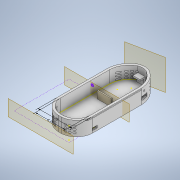
# Autodesk Inventor part: SkateBodyV2
Saved by Autodesk Inventor 2022 (Build 260153000, 153)
## iProperties
Created: 2024-10-16
Part Number: SkateBodyV2
Material: Generic
Document SubType Name: Modeling
Designer: karle
Density: 1 g/cm^3
Appearance: Default
Author: karle
## iProperties of the stored document SkateBodyV1_3DPrint.ipt
Created: 2024-10-16
Part Number: SkateBodyV1_3DPrint
Material: Generic
Document SubType Name: Modeling
Designer: karle
Density: 1 g/cm^3
Appearance: Default
Author: karle
Autodesk Inventor part; units mm, degrees
ref_plane "YZ Plane" through (0, 0, 0) normal (1, 0, 0) x (0, 1, 0)
ref_plane "XZ Plane" through (0, 0, 0) normal (0, 1, 0) x (-1, 0, 0)
ref_plane "XY Plane" through (0, 0, 0) normal (0, 0, 1) x (1, 0, 0)
sketch "Sketch1" plane through (0, 0, 0) normal (0, 1, 0) x (-1, 0, 0)
  line L0 (0, 0) -> (194.0278, 0) construction
  line L1 (194.0278, 0) -> (194.0278, -194.0278) construction
  line L2 (194.0278, -194.0278) -> (0, -194.0278) construction
  line L3 (0, -194.0278) -> (0, 0) construction
  constraints: 2 other
sketch "Sketch2" plane through (0, 0, 0) normal (0, 1, 0) x (-1, 0, 0)
  line L0 (-12.3873, -13.9985) -> (108.2627, -13.9985)
  line L1 (108.2627, -13.9985) -> (108.2627, -318.7985)
  line L2 (108.2627, -318.7985) -> (-12.3873, -318.7985)
  line L3 (-12.3873, -318.7985) -> (-12.3873, -13.9985)
  dimension "d1" = 120.65
  dimension "d2" = 304.8
  constraints: 8 end point, 2 parallel, 1 horizontal, 1 perpendicular
  measures "d1" distance of L1.end L2.end
  measures "d2" distance of L0.end L1.end
extrude "Extrusion1" add sketch "Sketch2" along normal blind 50.8
sketch "Sketch3" plane through (0, 50.8, 0) normal (0, 1, 0) x (1, 0, 0)
  line L0 (-108.2627, 318.7985) -> (-108.2627, 13.9985) projected
  line L1 (-108.2627, 13.9985) -> (12.3873, 13.9985) projected
  arc A0 (-108.2627, 68.9679) -> (-47.9377, 13.9985) centre (-49.7734, 72.5699) ccw
  line L2 (12.3873, 13.9985) -> (12.3873, 318.7985) projected
  arc A1 (-47.9377, 13.9985) -> (12.3873, 68.9679) centre (-44.4889, 70.7997) ccw
  line L3 (-108.2627, 68.9679) -> (-108.2627, 13.9985)
  line L4 (12.3873, 13.9985) -> (12.3873, 68.9679)
  line L5 (12.3873, 13.9985) -> (-108.2627, 13.9985)
  point P0 (0, 0)
  point P1 (-47.9377, 13.9985)
  point P2 (-41.0402, 13.9985)
  point P3 (-47.9377, 13.9985)
  point P4 (-51.609, 13.9985)
  constraints: 6 end point, 4 point on circle, 3 collinear, 2 centre point, 2 point on line, 1 midpoint
extrude "Extrusion2" cut sketch "Sketch3" against normal blind 50.8 contours A0 L1 L0 | A1 L2 L1
sketch "Sketch4" plane through (0, 50.8, 0) normal (0, 1, 0) x (1, 0, 0)
  line L0 (12.3873, 318.7985) -> (-108.2627, 318.7985) projected
  line L1 (-108.2627, 318.7985) -> (-108.2627, 13.9985) projected
  arc A0 (-47.9377, 318.7985) -> (-108.2627, 237.0618) centre (-27.9434, 240.9124) ccw
  line L2 (12.3873, 13.9985) -> (12.3873, 318.7985) projected
  arc A1 (12.3873, 237.0618) -> (-47.9377, 318.7985) centre (-69.3037, 239.9) ccw
  point P0 (0, 0)
  point P1 (-108.2627, 68.9679)
  point P2 (12.3873, 68.9679)
  point P3 (12.3873, 242.7382)
  point P4 (-108.2627, 244.763)
  constraints: 4 point on circle, 2 centre point, 2 point on line, 1 midpoint
extrude "Extrusion3" cut sketch "Sketch4" against normal blind 50.8 contours L2 A1 L0 | A0 L1 L0
sketch "Sketch5" plane through (0, 50.8, 0) normal (0, 1, 0) x (1, 0, 0)
  arc A0 (12.3873, 242.7382) -> (-47.9377, 318.7985) centre (-69.3037, 239.9) ccw projected
  arc A1 (-47.9377, 318.7985) -> (-108.2627, 244.763) centre (-27.9434, 240.9124) ccw projected
  arc A2 (-21.8713, 306.4706) -> (-76.8595, 304.7343) centre (-48.681, 283.9272) ccw
  arc A3 (-11.1383, 297.3306) -> (-85.2798, 297.2911) centre (-48.1933, 267.685) ccw
  point P0 (0, 0)
  point P1 (-72.79, 309.6054)
  point P2 (-66.5869, 311.4298)
  point P3 (-29.5638, 311.3298)
  constraints: 8 point on circle, 2 centre point
extrude "Extrusion4" cut sketch "Sketch5" against normal blind 50.8 contours A3 A1 A0
shell "Shell1" thickness 7.62 removed faces 1 at (-68.046, 50.8, -185.4897)
sketch "Sketch6" plane through (0, 50.8, 0) normal (0, 1, 0) x (1, 0, 0)
  arc A0 (-63.2764, 304.5535) -> (-100.6427, 244.5759) centre (-27.9434, 240.9124) ccw projected
  line L0 (-100.6427, 244.5759) -> (-100.6427, 69.2105) projected
  line L1 (4.7673, 69.095) -> (4.7673, 242.6026) projected
  arc A1 (4.7673, 242.6026) -> (-32.9147, 304.4729) centre (-69.3037, 239.9) ccw projected
  arc A2 (4.7673, 242.6026) -> (-32.9147, 304.4729) centre (-69.3037, 239.9) ccw projected
  line L2 (4.7673, 242.6026) -> (4.7673, 69.095) projected
  line L3 (-100.6427, 69.2105) -> (-100.6427, 244.5759) projected
  arc A3 (-63.2764, 304.5535) -> (-100.6427, 244.5759) centre (-27.9434, 240.9124) ccw projected
  arc A4 (-66.5869, 311.4298) -> (-108.2627, 244.763) centre (-27.9434, 240.9124) ccw projected
  line L4 (-108.2627, 244.763) -> (-108.2627, 68.9679) projected
  line L5 (12.3873, 68.9679) -> (12.3873, 242.7382) projected
  arc A5 (12.3873, 242.7382) -> (-29.5638, 311.3298) centre (-69.3037, 239.9) ccw projected
  line L6 (-108.2627, 244.763) -> (-108.2627, 68.9679) projected
  line L7 (-108.2627, 244.763) -> (-108.2627, 68.9679)
  arc A6 (-108.2627, 68.9679) -> (-51.609, 13.9985) centre (-49.7734, 72.5699) ccw projected
  arc A7 (-108.2627, 68.9679) -> (-54.2877, 13.9985) centre (-49.7646, 72.4238) ccw
  arc A8 (-41.0402, 13.9985) -> (12.3873, 68.9679) centre (-44.4889, 70.7997) ccw projected
  arc A9 (-54.2877, 13.9985) -> (12.3873, 68.9679) centre (-44.508, 70.0576) ccw
  line L8 (12.3873, 68.9679) -> (12.3873, 242.7382)
  arc A10 (12.3873, 242.7382) -> (-47.9377, 318.7985) centre (-69.3037, 239.9) ccw projected
  arc A11 (12.3873, 242.7382) -> (-34.4792, 308.438) centre (-68.917, 234.3062) ccw
  arc A12 (-34.4792, 308.438) -> (-72.79, 309.6054) centre (-54.5277, 279.7148) ccw projected
  arc A13 (-34.4792, 308.438) -> (-72.79, 309.6054) centre (-54.5277, 279.7148) ccw
  arc A14 (-47.9377, 318.7985) -> (-108.2627, 244.763) centre (-27.9434, 240.9124) ccw projected
  arc A15 (-72.79, 309.6054) -> (-108.2627, 244.763) centre (-34.0984, 246.3148) ccw
  arc A16 (-41.2796, 21.6185) -> (4.7673, 69.095) centre (-44.4889, 70.7997) ccw projected
  arc A17 (-100.6427, 69.2105) -> (-51.4855, 21.6185) centre (-49.7734, 72.5699) ccw projected
  arc A18 (-108.2627, 68.9679) -> (-51.609, 13.9985) centre (-49.7734, 72.5699) ccw projected
  arc A19 (-41.0402, 13.9985) -> (12.3873, 68.9679) centre (-44.4889, 70.7997) ccw projected
  arc A20 (-100.6427, 69.2105) -> (-51.4855, 21.6185) centre (-49.7734, 72.5699) ccw projected
  arc A21 (-41.2796, 21.6185) -> (4.7673, 69.095) centre (-44.4889, 70.7997) ccw projected
  line L9 (-41.2796, 21.6185) -> (-51.4855, 21.6185) projected
  line L10 (-51.609, 13.9985) -> (-41.0402, 13.9985) projected
  line L11 (-51.4855, 21.6185) -> (-41.2796, 21.6185) projected
  arc A22 (-32.9147, 304.4729) -> (-63.2764, 304.5535) centre (-48.1933, 267.685) ccw projected
  arc A23 (-29.5638, 311.3298) -> (-66.5869, 311.4298) centre (-48.1933, 267.685) ccw projected
  arc A24 (-32.9147, 304.4729) -> (-63.2764, 304.5535) centre (-48.1933, 267.685) ccw projected
  point P0 (0, 0)
  constraints: 10 point on circle, 5 centre point, 4 end point, 1 collinear, 1 vertical
extrude "Extrusion5" [suppressed]
sketch "Sketch7" plane through (0, 57.15, 0) normal (0, 1, 0) x (1, 0, 0)
  arc A0 (-7.9327, 246.4433) -> (-38.8697, 302.2099) centre (-81.9117, 241.8674) ccw projected
  arc A1 (-38.8697, 302.2099) -> (-68.687, 303.1821) centre (-54.5277, 279.7148) ccw projected
  arc A2 (-68.687, 303.1821) -> (-100.6427, 248.2322) centre (-28.0551, 242.7862) ccw projected
  line L0 (-100.6427, 69.2007) -> (-100.6427, 248.2322) projected
  line L1 (-7.9327, 246.4433) -> (-7.9327, 69.0971) projected
  arc A3 (-54.1879, 21.636) -> (-7.9327, 69.0971) centre (-57.1879, 70.8303) ccw projected
  arc A4 (-100.6427, 69.2007) -> (-54.1879, 21.636) centre (-49.7646, 72.4238) ccw projected
  point P0 (0, 0)
  point P1 (-54.337, 310.6675)
  point P2 (-100.6427, 21.6185)
  point P3 (-7.9327, 21.6185)
extrude "Extrusion6" [suppressed]
sketch "Sketch8" plane through (0, 50.8, 0) normal (0, 1, 0) x (1, 0, 0)
  arc A0 (-47.9889, 310.8895) -> (-100.6427, 244.5759) centre (-27.9434, 240.9124) ccw projected
  line L0 (-100.6427, 69.2105) -> (-100.6427, 244.5759) projected
  line L1 (-108.2627, 244.763) -> (-108.2627, 68.9679) projected
  arc A1 (-108.2627, 68.9679) -> (-51.609, 13.9985) centre (-49.7734, 72.5699) ccw projected
  arc A2 (-63.2764, 304.5535) -> (-100.6427, 244.5759) centre (-27.9434, 240.9124) ccw projected
  line L2 (-100.6427, 244.5759) -> (-100.6427, 69.2105) projected
  arc A3 (-100.6427, 69.2105) -> (-51.4855, 21.6185) centre (-49.7734, 72.5699) ccw projected
  arc A4 (-41.2796, 21.6185) -> (4.7673, 69.095) centre (-44.4889, 70.7997) ccw projected
  line L3 (4.7673, 69.095) -> (4.7673, 242.6026) projected
  arc A5 (4.7673, 242.6026) -> (-32.9147, 304.4729) centre (-69.3037, 239.9) ccw projected
  arc A6 (-41.0402, 13.9985) -> (12.3873, 68.9679) centre (-44.4889, 70.7997) ccw projected
  line L4 (12.3873, 68.9679) -> (12.3873, 242.7382) projected
  arc A7 (12.3873, 242.7382) -> (-47.9377, 318.7985) centre (-69.3037, 239.9) ccw projected
  arc A8 (-47.9377, 318.7985) -> (-108.2627, 244.763) centre (-27.9434, 240.9124) ccw projected
  arc A9 (4.7673, 242.6026) -> (-32.9147, 304.4729) centre (-69.3037, 239.9) ccw projected
  line L5 (4.7673, 242.6026) -> (4.7673, 69.095) projected
  arc A10 (-41.2796, 21.6185) -> (4.7673, 69.095) centre (-44.4889, 70.7997) ccw projected
  arc A11 (-100.6427, 69.2105) -> (-51.4855, 21.6185) centre (-49.7734, 72.5699) ccw projected
  line L6 (-100.6427, 69.2105) -> (-100.6427, 244.5759) projected
  arc A12 (-63.2764, 304.5535) -> (-100.6427, 244.5759) centre (-27.9434, 240.9124) ccw projected
  arc A13 (-66.5869, 311.4298) -> (-108.2627, 244.763) centre (-27.9434, 240.9124) ccw projected
  line L7 (-108.2627, 244.763) -> (-108.2627, 68.9679) projected
  arc A14 (-108.2627, 68.9679) -> (-51.609, 13.9985) centre (-49.7734, 72.5699) ccw projected
  arc A15 (-41.0402, 13.9985) -> (12.3873, 68.9679) centre (-44.4889, 70.7997) ccw projected
  line L8 (12.3873, 68.9679) -> (12.3873, 242.7382) projected
  arc A16 (12.3873, 242.7382) -> (-29.5638, 311.3298) centre (-69.3037, 239.9) ccw projected
  line L9 (-41.2796, 21.6185) -> (-51.4855, 21.6185) projected
  line L10 (-51.609, 13.9985) -> (-41.0402, 13.9985) projected
  line L11 (-51.4855, 21.6185) -> (-41.2796, 21.6185) projected
  arc A17 (-32.9147, 304.4729) -> (-63.2764, 304.5535) centre (-48.1933, 267.685) ccw projected
  arc A18 (-29.5638, 311.3298) -> (-66.5869, 311.4298) centre (-48.1933, 267.685) ccw projected
  arc A19 (-32.9147, 304.4729) -> (-63.2764, 304.5535) centre (-48.1933, 267.685) ccw projected
  point P0 (0, 0)
  point P1 (-68.687, 303.1821)
  point P2 (-54.2877, 13.9985)
  point P3 (-34.4792, 308.438)
  point P4 (-72.79, 309.6054)
  point P5 (-100.6427, 69.2105)
extrude "Extrusion7" [suppressed]
sketch "Sketch9" plane through (-100.6427, 7.62, -69.2007) normal (0, 1, 0) x (1, 0, 0)
  arc A0 (61.7729, 233.0092) -> (31.9557, 233.9815) centre (46.115, 210.5141) ccw projected
  arc A1 (31.9557, 233.9815) -> (0, 179.0316) centre (72.5876, 173.5855) ccw projected
  line L0 (0, 179.0316) -> (0, 0) projected
  arc A2 (0, 0) -> (46.4548, -47.5647) centre (50.8781, 3.2232) ccw projected
  arc A3 (46.4548, -47.5647) -> (92.71, -0.1035) centre (43.4547, 1.6296) ccw projected
  line L1 (92.71, -0.1035) -> (92.71, 177.2426) projected
  arc A4 (92.71, 177.2426) -> (61.7729, 233.0092) centre (18.731, 172.6667) ccw projected
  point P0 (100.6427, -69.2007)
extrude "Extrusion8" [suppressed]
sketch "Sketch10" plane through (-51.4855, 7.62, -21.6185) normal (0, 1, 0) x (1, 0, 0)
  line L0 (-25.4736, 153.821) -> (25.3264, 153.821)
  line L1 (25.3264, 153.821) -> (25.3264, 157.631)
  line L2 (25.3264, 157.631) -> (-25.4736, 157.631)
  line L3 (-25.4736, 157.631) -> (-25.4736, 153.821)
  arc A0 (21.9217, 289.7113) -> (-15.1014, 289.8112) centre (3.2922, 246.0665) ccw projected
  line L4 (3.2922, 293.521) -> (25.3264, 293.521)
  point P0 (51.4855, -21.6185)
  dimension "d28" = 50.8
  dimension "d29" = 3.81
  dimension "d30" = 135.89
  constraints: 10 end point, 2 horizontal, 2 parallel, 1 perpendicular, 1 point on circle, 1 tangent
  measures "d28" distance of L2.end L1.end
  measures "d29" distance of L1.end L0.end
  measures "d30" distance between parallel lines of L2 L4
extrude "Extrusion9" add sketch "Sketch10" along normal blind 25.4
sketch "Sketch11" plane through (-51.4855, 7.62, -21.6185) normal (0, 1, 0) x (1, 0, 0)
  arc A0 (21.9217, 289.7113) -> (-15.1014, 289.8112) centre (3.2922, 246.0665) ccw projected
  line L0 (3.2922, 293.521) -> (29.1501, 293.521)
  line L1 (-7.6984, 280.821) -> (17.7016, 280.821)
  line L2 (17.7016, 280.821) -> (17.7016, 275.741)
  line L3 (17.7016, 275.741) -> (-7.6984, 275.741)
  line L4 (-7.6984, 275.741) -> (-7.6984, 280.821)
  point P0 (51.4855, -21.6185)
  dimension "d33" = 25.4
  dimension "d34" = 5.08
  constraints: 10 end point, 2 horizontal, 2 parallel, 1 perpendicular, 1 point on circle, 1 tangent
  measures "d33" distance of L2.end L3.end
  measures "d34" distance of L1.end L2.end
extrude "Extrusion10" add sketch "Sketch11" along normal blind 25.4
sketch "Sketch12" plane through (-59.1839, 7.62, -297.3595) normal (0, 0, 1) x (1, 0, 0)
  line L0 (25.4, 0) -> (0, 0) projected
  line L1 (25.4, 0) -> (25.4, 25.4) projected
  line L2 (0, 25.4) -> (25.4, 25.4) projected
  line L3 (0, 0) -> (0, 25.4) projected
  line L4 (0, 25.4) -> (25.4, 25.4) projected
  line L5 (0, 0) -> (0, 25.4) projected
  line L6 (25.4, 25.4) -> (0, 25.4)
  line L7 (0, 25.4) -> (0, 20.32)
  line L8 (0, 20.32) -> (25.4, 20.32)
  line L9 (25.4, 20.32) -> (25.4, 25.4)
  point P0 (59.1839, -7.62)
  dimension "d38" = 5.08
  constraints: 8 end point, 2 parallel, 1 horizontal, 1 perpendicular, 1 point on line
  measures "d38" distance of L7.end L6.end
extrude "Extrusion11" add sketch "Sketch12" along normal blind 12.7 contours L8 L3 L2 L1
sketch "Sketch16" plane through (0, 50.8, 0) normal (0, 1, 0) x (1, 0, 0)
  point P0 (0, 0)
sketch "Sketch17" plane through (-51.4855, 7.62, -21.6185) normal (0, 1, 0) x (1, 0, 0)
  line L0 (-49.1572, 222.9574) -> (-49.1572, 47.592) projected
  arc A0 (-11.7909, 282.935) -> (-49.1572, 222.9574) centre (23.5421, 219.2939) ccw projected
  arc A1 (18.5708, 282.8544) -> (-11.7909, 282.935) centre (3.2922, 246.0665) ccw projected
  arc A2 (56.2528, 220.9841) -> (18.5708, 282.8544) centre (-17.8182, 218.2815) ccw projected
  line L1 (56.2528, 47.4765) -> (56.2528, 220.9841) projected
  arc A3 (10.2059, 0) -> (56.2528, 47.4765) centre (6.9966, 49.1811) ccw projected
  arc A4 (-49.1572, 47.592) -> (0, 0) centre (1.7121, 50.9514) ccw projected
  line L2 (0, 0) -> (10.2059, 0) projected
  point P0 (51.4855, -21.6185)
sketch "Sketch18" plane through (12.3873, 0, -68.9679) normal (1, 0, 0) x (0, 0, -1)
  line L0 (173.7703, 0) -> (173.7703, 50.8) projected
  line L1 (173.7703, 47.625) -> (-96.9224, 47.625)
  line L2 (-96.9224, 47.625) -> (-96.9224, 45.085)
  line L3 (-96.9224, 45.085) -> (173.7703, 45.085)
  line L4 (173.7703, 45.085) -> (173.7703, 47.625)
  line L5 (0, 50.8) -> (173.7703, 50.8) projected
  point P0 (-68.9679, 0)
  dimension "d63" = 2.54
  dimension "d64" = 3.175
  constraints: 8 end point, 2 parallel, 1 horizontal, 1 perpendicular, 1 point on line
  measures "d63" distance of L2.end L1.end
  measures "d64" distance between parallel lines of L5 L1
extrude "Extrusion12" cut sketch "Sketch18" against normal blind 3.81
sketch "Sketch19" plane through (-108.2627, 0, -68.9679) normal (-1, 0, 0) x (0, 0, 1)
  line L0 (-175.795, 50.8) -> (-175.795, 0) projected
  line L1 (-175.795, 44.45) -> (96.1328, 44.45)
  line L2 (96.1328, 44.45) -> (96.1328, 47.625)
  line L3 (96.1328, 47.625) -> (-175.795, 47.625)
  line L4 (-175.795, 47.625) -> (-175.795, 44.45)
  line L5 (-175.795, 50.8) -> (0, 50.8) projected
  point P0 (68.9679, 0)
  dimension "d67" = 3.175
  dimension "d68" = 3.175
  constraints: 8 end point, 2 parallel, 1 horizontal, 1 perpendicular, 1 point on line
  measures "d67" distance of L2.end L1.end
  measures "d68" distance between parallel lines of L5 L3
extrude "Extrusion13" cut sketch "Sketch19" against normal blind 3.81
sketch "Sketch23" plane through (12.3873, 0, -68.9679) normal (1, 0, 0) x (0, 0, -1)
  line L0 (1.6888, 7.874) -> (17.5638, 7.874)
  line L1 (17.5638, 7.874) -> (17.5638, 16.002)
  line L2 (17.5638, 16.002) -> (1.6888, 16.002)
  line L3 (1.6888, 16.002) -> (1.6888, 7.874)
  line L4 (0, 0) -> (173.7703, 0) projected
  point P0 (-68.9679, 0)
  dimension "d92" = 15.875
  dimension "d93" = 8.128
  dimension "d94" = 7.874
  constraints: 8 end point, 2 parallel, 1 horizontal, 1 perpendicular
  measures "d92" distance of L2.end L1.end
  measures "d93" distance of L1.end L0.end
  measures "d94" distance between parallel lines of L4 L0
extrude "Extrusion14" cut sketch "Sketch23" against normal blind 25.4
sketch "Sketch24" plane through (12.3873, 0, -68.9679) normal (1, 0, 0) x (0, 0, -1)
  line L0 (175.795, 44.45) -> (175.795, 0) projected
  line L1 (175.795, 24.384) -> (197.131, 24.384)
  line L2 (197.131, 24.384) -> (197.131, 12.7)
  line L3 (197.131, 12.7) -> (175.795, 12.7)
  line L4 (175.795, 12.7) -> (175.795, 24.384)
  line L5 (173.7703, 0) -> (242.3619, 0) projected
  point P0 (-68.9679, 0)
  dimension "d97" = 21.336
  dimension "d98" = 11.684
  dimension "d99" = 12.7
  constraints: 8 end point, 2 parallel, 1 horizontal, 1 perpendicular, 1 point on line
  measures "d97" distance of L2.end L3.end
  measures "d98" distance of L1.end L2.end
  measures "d99" distance between parallel lines of L5 L3
extrude "Extrusion15" cut sketch "Sketch24" against normal blind 25.4
sketch "Sketch25" plane through (12.3873, 0, -68.9679) normal (1, 0, 0) x (0, 0, -1)
  circle A0 centre (184.1171, 38.1) radius 2.794
  line L0 (242.3619, 50.8) -> (173.7703, 50.8) projected
  point P0 (-68.9679, 0)
  dimension "d102" = 5.588
  dimension "d103" = 12.7
  constraints: 1 centre point
  measures "d102" diameter of A0
  measures "d103" distance from line of L0 A0.centre
extrude "Extrusion16" cut sketch "Sketch25" against normal blind 25.4
ref_plane "Work Plane1" through (-66.5869, 50.8, -311.4298) normal (0.1964, 0, 0.9805) x (0, -1, 0)
sketch "Sketch26" plane through (-66.5869, 50.8, -311.4298) normal (0.1964, 0, 0.9805) x (0, -1, 0)
  point P0 (50.8, 4.1311)
ref_plane "Work Plane2" through (-76.9591, 33.02, -175.4395) normal (0, 0, 1) x (1, 0, 0)
sketch "Sketch27" plane through (-76.9591, 33.02, -175.4395) normal (0, 0, 1) x (1, 0, 0)
  circle A0 centre (-17.0655, 8.0994) radius 4.1905
  point P0 (76.9591, -33.02)
  constraints: 1 centre point
ref_plane "Work Plane3" through (-76.9591, 33.02, 27.7605) normal (0, 0, 1) x (1, 0, 0)
sketch "Sketch28" plane through (-76.9591, 33.02, 27.7605) normal (0, 0, 1) x (1, 0, 0)
  line L0 (-27.4936, 11.43) -> (-31.3036, 11.43) construction
  line L1 (-31.3036, -33.02) -> (-31.3036, 11.43) construction
  line L2 (25.3501, -33.02) -> (-31.3036, -33.02) construction
  line L3 (25.3501, 17.78) -> (25.3501, -33.02) construction
  line L4 (-31.3036, 17.78) -> (25.3501, 17.78) construction
  line L5 (-31.3036, 14.605) -> (-31.3036, 17.78) construction
  line L6 (-31.3036, 14.605) -> (-27.4936, 14.605) construction
  line L7 (-27.4936, 14.605) -> (-27.4936, 11.43) construction
  line L8 (85.5364, 14.605) -> (89.3464, 14.605) construction
  line L9 (89.3464, 17.78) -> (89.3464, 14.605) construction
  line L10 (35.9189, 17.78) -> (89.3464, 17.78) construction
  line L11 (35.9189, -33.02) -> (35.9189, 17.78) construction
  line L12 (89.3464, -33.02) -> (35.9189, -33.02) construction
  line L13 (89.3464, 12.065) -> (89.3464, -33.02) construction
  line L14 (89.3464, 12.065) -> (85.5364, 12.065) construction
  line L15 (85.5364, 12.065) -> (85.5364, 14.605) construction
  line L16 (35.9189, -33.02) -> (35.9189, 17.78) construction
  line L17 (25.3501, 17.78) -> (35.9189, 17.78) construction
  line L18 (25.3501, 17.78) -> (25.3501, -33.02) construction
  line L19 (25.3501, -33.02) -> (35.9189, -33.02) construction
  line L20 (47.3953, 17.78) -> (10.3722, 17.78) construction
  line L21 (30.6345, 17.78) -> (30.6345, -33.8757) construction
  line L22 (10.3722, -33.02) -> (47.3953, -33.02) construction
  circle A0 centre (-17.8897, -0.2155) radius 3.2384
  circle A1 centre (79.1588, -0.2155) radius 3.2384
  circle A2 centre (-17.8897, -10.3755) radius 3.2384
  circle A3 centre (-17.8897, -20.5355) radius 3.2384
  circle A4 centre (-7.7297, -0.2155) radius 3.2384
  circle A5 centre (-7.7297, -10.3755) radius 3.2384
  circle A6 centre (-7.7297, -20.5355) radius 3.2384
  circle A7 centre (2.4303, -0.2155) radius 3.2384
  circle A8 centre (2.4303, -10.3755) radius 3.2384
  circle A9 centre (2.4303, -20.5355) radius 3.2384
  circle A10 centre (12.5903, -0.2155) radius 3.2384
  circle A11 centre (12.5903, -10.3755) radius 3.2384
  circle A12 centre (12.5903, -20.5355) radius 3.2384
  circle A13 centre (79.1588, -0.2155) radius 3.2384
  circle A14 centre (79.1588, -10.3755) radius 3.2384
  circle A15 centre (79.1588, -20.5355) radius 3.2384
  circle A16 centre (68.9988, -0.2155) radius 3.2384
  circle A17 centre (68.9988, -10.3755) radius 3.2384
  circle A18 centre (68.9988, -20.5355) radius 3.2384
  circle A19 centre (58.8388, -0.2155) radius 3.2384
  circle A20 centre (58.8388, -10.3755) radius 3.2384
  circle A21 centre (58.8388, -20.5355) radius 3.2384
  circle A22 centre (48.6788, -0.2155) radius 3.2384
  circle A23 centre (48.6788, -10.3755) radius 3.2384
  circle A24 centre (48.6788, -20.5355) radius 3.2384
  point P0 (76.9591, -33.02)
  point P1 (-9.8875, -0.2155)
  point P2 (71.1565, -0.2155)
  dimension "d109" = 10.16
  dimension "d112" = 10.16
  constraints: 25 centre point, 14 symmetric about line, 2 end point, 1 horizontal, 1 perpendicular, 1 point on line, 1 vertical, 35 other
  measures "d109" distance of A0.centre A2.centre
  measures "d112" distance of A0.centre A4.centre
extrude "Extrusion17" cut sketch "Sketch28" against normal blind 355.6 contours A0 | A2 | A3 | A4 | A5 | A6 | A7 | A8 | A9 | A10 | A11 | A12 | A16 | A17 | A18 | A19 | A20 | A21 | A22 | A23 | A24
sketch "Sketch29" plane through (-66.5869, 50.8, -311.4298) normal (0.1964, 0, 0.9805) x (0, -1, 0)
  point P0 (50.8, 4.1311)
sketch "Sketch30" plane through (-51.4855, 7.62, -21.6185) normal (0, 1, 0) x (1, 0, 0)
  line L0 (-7.6984, 275.741) -> (-7.6984, 280.821) projected
  line L1 (-7.6984, 280.821) -> (17.7016, 280.821) projected
  line L2 (17.7016, 280.821) -> (17.7016, 275.741) projected
  line L3 (17.7016, 275.741) -> (-7.6984, 275.741) projected
  line L4 (25.3264, 153.821) -> (-25.4736, 153.821) projected
  line L5 (-25.4736, 153.821) -> (-25.4736, 157.631) projected
  line L6 (-25.4736, 157.631) -> (25.3264, 157.631) projected
  line L7 (25.3264, 157.631) -> (25.3264, 153.821) projected
  arc A0 (18.5708, 282.8544) -> (-11.7909, 282.935) centre (3.2922, 246.0665) ccw projected
  arc A1 (-11.7909, 282.935) -> (-49.1572, 222.9574) centre (23.5421, 219.2939) ccw projected
  line L8 (-49.1572, 222.9574) -> (-49.1572, 47.592) projected
  arc A2 (-49.1572, 47.592) -> (0, 0) centre (1.7121, 50.9514) ccw projected
  line L9 (0, 0) -> (10.2059, 0) projected
  arc A3 (10.2059, 0) -> (56.2528, 47.4765) centre (6.9966, 49.1811) ccw projected
  line L10 (56.2528, 47.4765) -> (56.2528, 220.9841) projected
  arc A4 (56.2528, 220.9841) -> (18.5708, 282.8544) centre (-17.8182, 218.2815) ccw projected
  line L11 (-25.4736, 153.821) -> (-25.4736, 157.631) projected
  line L12 (25.3264, 153.821) -> (-25.4736, 153.821) projected
  line L13 (-25.4736, 157.631) -> (25.3264, 157.631)
  line L14 (25.3264, 157.631) -> (25.3264, 153.821)
  line L15 (25.3264, 153.821) -> (-25.4736, 153.821)
  line L16 (-25.4736, 153.821) -> (-25.4736, 157.631)
  point P0 (51.4855, -21.6185)
  constraints: 8 end point, 2 parallel, 1 horizontal, 1 perpendicular
extrude "Extrusion18" add sketch "Sketch30" along normal blind 25.4 contours L4 L5 L6 L7
body "Solid1"
